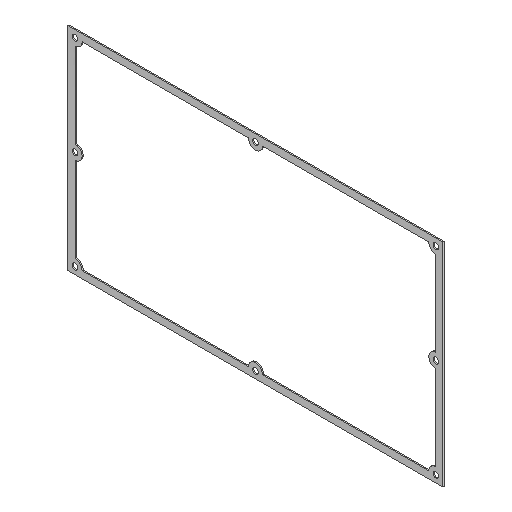
# Autodesk Inventor part: Empaque
Saved by Autodesk Inventor 2025.2 (Build 292293000, 293)
## iProperties
Created: 2025-08-05
Part Number: Empaque
Material: Generic
Document SubType Name: Modeling
Designer: Compa
Density: 1 g/cm^3
Appearance: Default
Author: Compa
Autodesk Inventor part; units mm, degrees
ref_plane "YZ Plane" through (0, 0, 0) normal (1, 0, 0) x (0, 1, 0)
ref_plane "XZ Plane" through (0, 0, 0) normal (0, 1, 0) x (-1, 0, 0)
ref_plane "XY Plane" through (0, 0, 0) normal (0, 0, 1) x (1, 0, 0)
sketch "Sketch1" plane through (0, 0, 0) normal (0, 0, 1) x (1, 0, 0)
  line L0 (0, 0) -> (265, 0)
  line L1 (265, 0) -> (265, -150)
  line L2 (265, -150) -> (0, -150)
  line L3 (0, -150) -> (0, 0)
  line L4 (260, -5) -> (5, -5)
  line L5 (5, -5) -> (5, -145)
  line L6 (5, -145) -> (260, -145)
  line L7 (260, -145) -> (260, -5)
  circle A0 centre (5, -5) radius 5
  circle A1 centre (260, -5) radius 5
  circle A2 centre (260, -145) radius 5
  circle A3 centre (5, -145) radius 5
  line L8 (5, -5) -> (5, -75)
  circle A4 centre (5, -75) radius 5
  line L9 (260, -5) -> (260, -75)
  circle A5 centre (260, -75) radius 5
  line L10 (5, -5) -> (132.5, -5)
  circle A6 centre (132.5, -5) radius 5
  line L11 (5, -145) -> (132.5, -145)
  circle A7 centre (132.5, -145) radius 5
  circle A8 centre (5, -5) radius 2.05
  circle A9 centre (5, -75) radius 2.05
  circle A10 centre (5, -145) radius 2.05
  circle A11 centre (132.5, -145) radius 2.05
  circle A12 centre (260, -145) radius 2.05
  circle A13 centre (260, -75) radius 2.05
  circle A14 centre (260, -5) radius 2.05
  circle A15 centre (132.5, -5) radius 2.05
  point P0 (5, -140)
  point P1 (5, -80)
  point P2 (5, -70)
  point P3 (5, -10)
  point P4 (10, -5)
  point P5 (127.5, -5)
  point P6 (137.5, -5)
  point P7 (255, -5)
  point P8 (260, -10)
  point P9 (260, -70)
  point P10 (260, -80)
  point P11 (260, -140)
  point P12 (255, -145)
  point P13 (137.5, -145)
  point P14 (127.5, -145)
  point P15 (10, -145)
  dimension "d0" = 265
  dimension "d1" = 150
  dimension "d2" = 5
  dimension "d3" = 10
  dimension "d4" = 10
  dimension "d5" = 10
  dimension "d6" = 10
  dimension "d7" = 70
  dimension "d8" = 10
  dimension "d9" = 70
  dimension "d10" = 10
  dimension "d11" = 127.5
  dimension "d12" = 10
  dimension "d13" = 127.5
  dimension "d14" = 10
  dimension "d15" = 4.1
  dimension "d16" = 4.1
  dimension "d17" = 4.1
  dimension "d18" = 4.1
  dimension "d19" = 4.1
  dimension "d20" = 4.1
  dimension "d21" = 4.1
  dimension "d22" = 4.1
  constraints: 24 end point, 16 centre point, 16 coincident, 6 perpendicular, 4 midpoint, 1 horizontal, 3 other
  measures "d0" distance of L0.start L0.end
  measures "d1" distance of L0.end L1.end
  measures "d2" distance between parallel lines of L0 L4
  measures "d3" diameter of A0
  measures "d4" diameter of A1
  measures "d5" diameter of A2
  measures "d6" diameter of A3
  measures "d7" distance of L8.start L8.end
  measures "d8" diameter of A4
  measures "d9" distance of L9.start L9.end
  measures "d10" diameter of A5
  measures "d11" distance of L8.start L10.end
  measures "d12" diameter of A6
  measures "d13" distance of L11.start L11.end
  measures "d14" diameter of A7
  measures "d15" diameter of A8
  measures "d16" diameter of A9
  measures "d17" diameter of A10
  measures "d18" diameter of A11
  measures "d19" diameter of A12
  measures "d20" diameter of A13
  measures "d21" diameter of A14
  measures "d22" diameter of A15
extrude "Extrusion1" add sketch "Sketch1" along normal blind 0.8 contours L0 A0 L3 | L0 A6 L4 A0 | A0 L4 A8 L5 | A0 L5 A4 L3 | L0 A1 L4 A6 | A6 L4 A15 | A0 L5 A8 L4 | A4 L5 A3 L3 | A4 L5 A9 | L0 L1 A1 | A1 L7 A14 L4 | A6 L4 A15 | A3 L2 L3 | A3 L5 A10 L6 | A4 L5 A9 | L1 A5 L7 A1 | L4 A14 L7 A1 | A3 L6 A10 L5 | A3 L6 A7 L2 | A5 L7 A13 | L1 A2 L7 A5 | A7 L6 A2 L2 | A7 L6 A11 | A2 L6 A12 L7 | L1 L2 A2 | L7 A13 A5 | A7 L6 A11 | L7 A12 L6 A2
body "Solid1"
